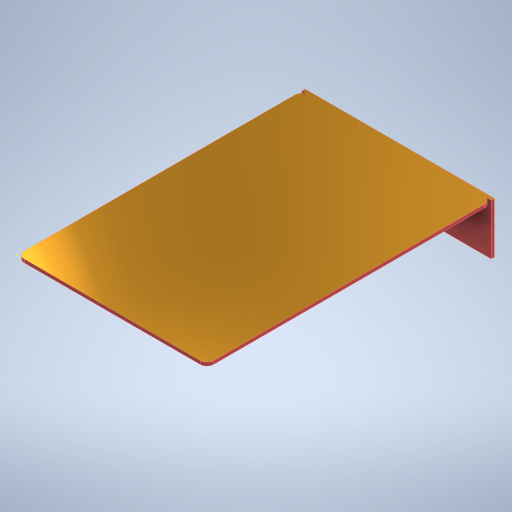
# Autodesk Inventor part: cover
Saved by Autodesk Inventor 2023 (Build 270158000, 158)
## iProperties
Created: 2023-01-13
Part Number: cover
Material: Generic
Document SubType Name: Modeling
Designer: zhanj390
Density: 1 g/cm^3
Appearance: Orange-Red
Author: zhanj390
Autodesk Inventor part; units mm, degrees
ref_plane "YZ Plane" through (0, 0, 0) normal (1, 0, 0) x (0, 1, 0)
ref_plane "XZ Plane" through (0, 0, 0) normal (0, 1, 0) x (-1, 0, 0)
sketch "Sketch1" plane through (0, 0, 0) normal (0, 1, 0) x (-1, 0, 0)
  line L0 (0, 0) -> (-56, 0)
  line L1 (-56, 0) -> (-56, -84)
  line L2 (-56, -84) -> (0, -84)
  line L3 (0, -84) -> (0, 0)
  point P0 (-28, -84)
  dimension "d0" = 56
  dimension "d1" = 84
  constraints: 8 end point, 2 parallel, 1 horizontal, 1 midpoint, 1 perpendicular
  measures "d0" distance of L1.end L2.end
  measures "d1" distance from line of point (-28, -84) L0
extrude "Extrusion1" add sketch "Sketch1" along normal blind 1
fillet "Fillet1" radius 2 1 edges at (0, 0.5, 0)
fillet "Fillet2" radius 2 1 edges at (56, 0.5, 0)
fillet "Fillet3" radius 2 1 edges at (56, 0.5, -84)
fillet "Fillet4" radius 2 1 edges at (0, 0.5, -84)
sketch "Sketch2" plane through (0, 1, 0) normal (0, 1, 0) x (1, 0, 0)
  point P0 (0, 0)
ref_plane "Work Plane1" through (54, 0, -84) normal (0, 0, -1) x (-1, 0, 0)
sketch "Sketch3" plane through (54, 0, -84) normal (0, 0, -1) x (-1, 0, 0)
  line L0 (-2, 1) -> (0, 1) projected
  line L1 (-2, 1) -> (54, 1)
  line L2 (54, 1) -> (54, -14)
  line L3 (54, -14) -> (-2, -14)
  line L4 (-2, -14) -> (-2, 1)
  point P0 (54, 0)
  dimension "d9" = 0
  dimension "d10" = 15
  constraints: 8 end point, 2 parallel, 1 horizontal, 1 perpendicular
  measures "d9" distance from line of point (54, 0) L2
  measures "d10" distance between parallel lines of L1 L3
extrude "Extrusion2" add sketch "Sketch3" along normal blind 1
body "Solid1"
